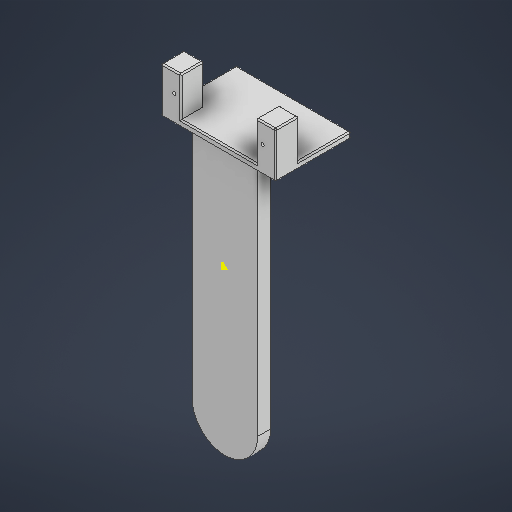
# Autodesk Inventor part: L1
Saved by Autodesk Inventor 2026 (Build 300175000, 175)
## iProperties
Created: 2026-02-13
Part Number: L1
Material: Generisch
Document SubType Name: Modeling
Designer: Jakob Dorninger
Density: 1 g/cm^3
Appearance: Vorgabe
Author: Jakob Dorninger
Autodesk Inventor part; units mm, degrees
ref_plane "YZ Plane" through (0, 0, 0) normal (1, 0, 0) x (0, 1, 0)
ref_plane "XZ Plane" through (0, 0, 0) normal (0, 1, 0) x (-1, 0, 0)
ref_plane "XY Plane" through (0, 0, 0) normal (0, 0, 1) x (1, 0, 0)
sketch "Skizze1" plane through (0, 0, 0) normal (0, 1, 0) x (-1, 0, 0)
  line L0 (-10, -50) -> (10, -50)
  line L1 (10, -50) -> (10, 50)
  line L2 (10, 50) -> (-10, 50)
  line L3 (-10, 50) -> (-10, -50)
  line L4 (-10, -50) -> (10, 50) construction
  line L5 (10, -50) -> (-10, 50) construction
  point P0 (0, 0)
  dimension "d0" = 20
  dimension "d1" = 100
  constraints: 12 end point, 2 midpoint, 2 parallel, 1 horizontal, 1 perpendicular
  measures "d0" distance of L2.end L1.end
  measures "d1" distance of L2.end L0.start
extrude "Extrusion1" add sketch "Skizze1" along normal blind 4
fillet "Rundung1" radius 10 4 edges at (10, 2, -50) (-10, 2, -50) (10, 2, 50) (-10, 2, 50)
sketch "Skizze2" plane through (0, 0, 0) normal (0, -1, 0) x (1, 0, 0)
  point P0 (0, 0)
sketch "Skizze3" plane through (0, 0, 0) normal (0, -1, 0) x (1, 0, 0)
  line L0 (-17.5, 34) -> (-17.5, 46)
  line L1 (17.5, 46) -> (17.5, 34)
  line L2 (-11.5, 46) -> (-11.5, 34)
  line L3 (11.5, 46) -> (11.5, 34)
  line L4 (0, -70) -> (0, 70) projected
  line L5 (-17.5, 46) -> (-11.5, 46)
  line L6 (11.5, 46) -> (17.5, 46)
  line L7 (17.5, 34) -> (11.5, 34)
  line L8 (-11.5, 34) -> (-17.5, 34)
  point P0 (0, 0)
  point P1 (0, 34)
  point P2 (11.5, 40)
  point P3 (17.5, 40)
  point P4 (-11.5, 40)
  point P5 (-17.5, 40)
  point P6 (14.5, 34)
  point P7 (-14.5, 34)
  dimension "d6" = 12
  dimension "d7" = 35
  dimension "d11" = 23
  dimension "d12" = 34
  dimension "d13" = 6
  constraints: 16 end point, 6 horizontal alignment, 6 midpoint, 6 perpendicular, 5 parallel, 2 horizontal, 1 point on line, 1 vertical alignment, 1 other
  measures "d6" distance of L0.start L0.end
  measures "d7" distance between parallel lines of L1 L0
  measures "d11" distance between parallel lines of L3 L2
  measures "d12" distance of point (0, 0) point (0, 34)
  measures "d13" distance between parallel lines of L1 L3
sketch "Skizze4" plane through (0, 0, 0) normal (0, -1, 0) x (1, 0, 0)
  arc A0 (10, 40) -> (-10, 40) centre (0, 40) ccw projected
  line L0 (-11.5, 34) -> (-17.5, 34) projected
  line L1 (11.5, 46) -> (11.5, 34) projected
  line L2 (-11.5, 34) -> (11.5, 34)
  line L3 (11.5, 34) -> (11.5, 53)
  line L4 (11.5, 53) -> (-11.5, 53)
  line L5 (-11.5, 53) -> (-11.5, 34)
  point P0 (0, 0)
  dimension "d14" = 19
  constraints: 8 end point, 2 parallel, 1 horizontal, 1 perpendicular, 1 vertical alignment
  measures "d14" distance between parallel lines of L2 L4
extrude "Extrusion2" cut sketch "Skizze4" against normal blind 4
extrude "Extrusion3" add sketch "Skizze3" along normal blind 2 and the other way blind 5
sketch "Skizze5" plane through (0, 0, 0) normal (0, -1, 0) x (1, 0, 0)
  line L0 (-17.5, 34) -> (-11.5, 34) projected
  line L1 (11.5, 34) -> (17.5, 34) projected
  line L2 (-17.5, 34) -> (17.5, 34)
  line L3 (17.5, 34) -> (17.5, 32)
  line L4 (17.5, 32) -> (-17.5, 32)
  line L5 (-17.5, 32) -> (-17.5, 34)
  point P0 (0, 0)
  dimension "d21" = 2
  constraints: 8 end point, 2 parallel, 1 horizontal, 1 perpendicular, 1 vertical alignment
  measures "d21" distance of L2.end L3.end
extrude "Extrusion4" add sketch "Skizze5" along normal blind 2 and the other way blind 21
fillet "Rundung2" radius 1 4 edges at (10, 2, 32) (0, 0, 32) (0, 4, 32) (-10, 2, 32)
chamfer "Fasen1" distance 0.4 angle 45 7 edges at (-11.5, -2, 40) (-11.5, 1.5, 46) (11.5, -2, 40) (11.5, 1.5, 46) (-11.5, 5, 40) (11.5, 5, 40) (0, -2, 34)
fillet "Rundung3" radius 0.4 19 edges at (-14.7, -2, 46) (-14.7, 5, 46) (-17.5, 1.5, 46) (14.7, 5, 46) (14.7, -2, 46) (17.5, 1.5, 46) (17.5, -2, 39) (17.5, 5, 40) (17.5, 13, 34) (17.5, 9.5, 32) (0, 21, 34) (0, -2, 32) (-17.5, 13, 34) (-17.5, 21, 33) (-17.5, 9.5, 32) (-17.5, -2, 39) (-17.5, 5, 40) (17.5, 21, 33) (0, 21, 32)
sketch "Skizze6" plane through (0, -2, 0) normal (0, -1, 0) x (1, 0, 0)
  line L0 (-17.1, 45.6) -> (-11.9, 45.6) projected
  line L1 (11.9, 45.6) -> (17.1, 45.6) projected
  line L2 (11.5, 34) -> (-11.5, 34) projected
  line L3 (0, -69.2) -> (0, 65.2) projected
  point P0 (0, 0)
  point P1 (-13.5, 40)
  point P2 (13.5, 40)
  dimension "d31" = 6
  dimension "d32" = 27
  constraints: 1 horizontal alignment, 1 symmetric about line
  measures "d31" distance from line of L2 point (-13.5, 40)
  measures "d32" distance of point (13.5, 40) point (-13.5, 40)
hole "Bohrung1" at (-13.5, -2, 40) at (13.5, -2, 40) direction (0, 1, 0) diameter 1 end through all
